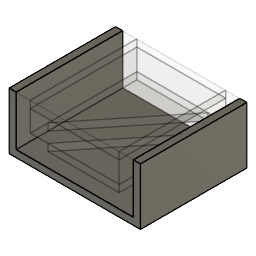
V4.3 (Autodesk Fusion 360 design; units mm, degrees)
part number: 2026-06-11-15-33-25-034
part number: 2026-06-11-15-44-55-864
part number: 2026-06-11-15-46-27-976
part number: 2026-06-11-15-51-44-010
part number: 2026-06-11-15-55-50-120
part number: 2026-06-18-15-30-37-176
part number: 2026-06-18-15-32-28-771
part number: 2026-06-18-15-36-27-577
part number: 2026-06-18-15-36-38-430
part number: 2026-06-18-15-43-19-432
part number: 2026-06-18-15-44-30-441
Autodesk Fusion 360 part; units mm, degrees
sketch "Esquisse5" plane through (0, 0, 0) normal (0, 0, 1) x (1, 0, 0)
  line L0 (0, 0) -> (37, 0)
  line L1 (37, 0) -> (37, 30)
  line L2 (37, 30) -> (0, 30)
  line L3 (0, 30) -> (0, 0)
  line L4 (0, 30) -> (2, 30)
  line L5 (2, 30) -> (2, 0)
  line L6 (2, 0) -> (0, 0)
  line L7 (0, 0) -> (0, 30)
  dimension "d48" = 37
  dimension "d49" = 30
  dimension "d50" = 2
  dimension "d51" = 30
  constraint horizontal L0
  constraint vertical L1
  constraint horizontal L2
  constraint vertical L3
  constraint coincident L0.start L3.end
  constraint horizontal L4
  constraint vertical L5
  constraint horizontal L6
  constraint vertical L7
  measures "d48" distance of L0.start L0.end
  measures "d49" distance of L0.start L2.end
  measures "d50" distance of L2.end L4.end
  measures "d51" distance of L2.end L0.start
extrude "Extrusion1" add sketch "Esquisse5" along normal blind 2 contours L0 L1 L2 L5 makes body 1 in component "Shield"
sketch "Esquisse1" plane through (0, 0, 0) normal (0, 0, 1) x (1, 0, 0) in component "Shield"
  line L0 (2, 30) -> (0, 30)
  line L1 (0, 30) -> (0, 0)
  line L2 (0, 0) -> (2, 0)
  line L3 (2, 0) -> (2, 30)
  line L4 (35, 30) -> (37, 30)
  line L5 (37, 30) -> (37, 0)
  line L6 (37, 0) -> (35, 0)
  line L7 (35, 0) -> (35, 30)
  point P0 (37, 0)
  dimension "d54" = 2
  dimension "d55" = 30
  dimension "d56" = 2
  dimension "d57" = 30
  constraint horizontal L0
  constraint vertical L1
  constraint horizontal L2
  constraint vertical L3
  constraint horizontal L4
  constraint vertical L5
  constraint horizontal L6
  constraint vertical L7
  constraint coincident L5 P0
  measures "d54" distance of L0.start L0.end
  measures "d55" distance of L0.start L2.end
  measures "d56" distance of L4.start L4.end
  measures "d57" distance of L4.start L6.end
extrude "Extrusion2" add sketch "Esquisse1" along normal blind 16 bodies 1 in component "Shield"
sketch "Esquisse2" plane through (0, 0, 2) normal (0, 0, 1) x (-1, 0, 0) in component "Shield"
  line L0 (-2, -30) -> (-2, 0)
  line L1 (-2, 0) -> (-35, 0)
  line L2 (-35, 0) -> (-35, -30)
  line L3 (-35, -30) -> (-2, -30)
sketch "Esquisse1 (2)" plane through (0, 0, 2) normal (0, 0, 1) x (-1, 0, 0) in component "Support"
  line L0 (-2, 0) -> (-6, 0)
  line L1 (-6, 0) -> (-6, -30)
  line L2 (-6, -30) -> (-2, -30)
  line L3 (-2, -30) -> (-2, 0)
  line L4 (-35, -30) -> (-31, -30)
  line L5 (-31, -30) -> (-31, 0)
  line L6 (-31, 0) -> (-35, 0)
  line L7 (-35, 0) -> (-35, -30)
  point P0 (-37, 0)
  dimension "d60" = 4
  dimension "d61" = 4
  dimension "d62" = 30
  dimension "d86" = 2
  dimension "d87" = 2
  constraint horizontal L0
  constraint vertical L1
  constraint horizontal L2
  constraint vertical L3
  constraint horizontal L4
  constraint vertical L5
  constraint horizontal L6
  constraint vertical L7
  measures "d60" distance of L0.start L0.end
  measures "d61" distance of L4.start L4.end
  measures "d62" distance of L4.start L6.end
  measures "d86" distance of origin L0.start
  measures "d87" distance of L6.end P0
extrude "Extrusion1'" add sketch "Esquisse1 (2)" along normal blind 14 separate body makes body 2 at (2, 20, 6.6667) makes body 3 at (35, 10, 6.6667) in component "Support"
extrude "Extrusion2'" add sketch "Esquisse2" along normal blind 4 bodies 2 3 in component "Support"
sketch "Esquisse2 (2)" plane through (0, 0, 6) normal (0, 0, 1) x (-1, 0, 0) in component "Support"
  line L0 (-6, -30) -> (-6, 0)
  line L1 (-6, 0) -> (-31, 0)
  line L2 (-31, 0) -> (-31, -30)
  line L3 (-31, -30) -> (-6, -30)
sketch "Esquisse1 (3)" plane through (0, 0, 6) normal (0, 0, 1) x (-1, 0, 0) in component "Capteur2"
  line L0 (-6, -5) -> (-26, -30)
  line L1 (-6, -30) -> (-6, 0)
  line L2 (-31, -30) -> (-6, -30)
  point P0 (-6, -30)
  point P1 (-6, 0)
  dimension "d67" = 20
  dimension "d69" = 5
  constraint coincident L0.start L1
  constraint coincident L0.end L2
  measures "d67" distance of L0.end P0
  measures "d69" distance of L0.start L1.end
extrude "Extrusion1''" add sketch "Esquisse1 (3)" along normal blind 2 separate body makes body 4 in component "Capteur2"
sketch "Esquisse2 (3)" plane through (0, 0, 6) normal (0, 0, 1) x (-1, 0, 0) in component "Capteur2"
  line L0 (-11, 0) -> (-31, -25)
  line L1 (-31, 0) -> (-31, -30)
  line L2 (-6, 0) -> (-31, 0)
  point P0 (-31, 0)
  point P1 (-31, -30)
  dimension "d72" = 20
  dimension "d73" = 5
  constraint coincident L0.end L1
  constraint coincident L0.start L2
  measures "d72" distance of L0.start P0
  measures "d73" vertical distance of L0.end P1
extrude "Extrusion1'''" add sketch "Esquisse2 (3)" along normal blind 2 separate body makes body 5 in component "Capteur1"
extrude "Extrusion3" add sketch "Esquisse2 (2)" along normal blind 2 bodies 2 in component "Support"
copy_body "CopierCollerCorps1" bodies 5 4 makes body 6 makes body 7 in component "Support"
combine "Combiner1" operation cut target body 2 tool bodies 6 7 in component "Support"
extrude "Extrusion1''''" add 1 faces at (21, 20, 8) along direction (0, 0, 1) blind 6 separate body on bodies 2 makes body 8 in component "Mousse (1)"
extrude "Extrusion2''" add 1 faces at (24.3333, 8.3333, 8) along direction (0, 0, 1) blind 6 on bodies 5 bodies 8 in component "Mousse (1)"
extrude "Extrusion3'" add 1 faces at (12.6667, 21.6667, 8) along direction (0, 0, 1) blind 6 on bodies 4 bodies 8 in component "Mousse (1)"
extrude "Extrusion1'''''" add 1 faces at (22.6667, 10, 14) along direction (0, 0, 1) blind 2 separate body on bodies 8 makes body 9 in component "plateau (1)"
sketch "Esquisse1 (4)" plane through (0, 0, 6) normal (0, 0, 1) x (-1, 0, 0) in component "trianglee_1"
  line L0 (-16, 0) -> (-16, -30)
  line L1 (-16, -30) -> (-6, -30)
  line L2 (-6, -30) -> (-6, 0)
  line L3 (-6, 0) -> (-16, 0)
  spline S0 degree 5 poles (-6, 0) (-6.4, -1) (-7.2, -3) (-8.4, -6) (-10, -10) (-12, -15) (-13.6, -19) (-14.8, -22) (-15.6, -24) (-16, -25) knots 0 0 0 0 0 0 0.2 0.4 0.6 0.8 1 1 1 1 1 1
  dimension "d33" = 5
  dimension "d47" = 20
  constraint coincident L3 L2.end
  constraint coincident L0 S0.end
  measures "d33" distance of L0.end S0.end
extrude "Extrusion1''''''" [rolled back] along distance 2 taper angle 0 in component "trianglee_1"
sketch "Esquisse1 (5)" plane through (0, 0, 6) normal (0, 0, 1) x (-1, 0, 0) in component "triangle_2"
  line L0 (-16, 0) -> (-16, -30)
  line L1 (-16, -30) -> (-6, -30)
  line L2 (-6, -30) -> (-6, 0)
  line L3 (-6, 0) -> (-16, 0)
  spline S0 degree 5 poles (-6, -5) (-6.4, -6) (-7.2, -8) (-8.4, -11) (-10, -15) (-12, -20) (-13.6, -24) (-14.8, -27) (-15.6, -29) (-16, -30) knots 0 0 0 0 0 0 0.2 0.4 0.6 0.8 1 1 1 1 1 1
  dimension "d37" = 5
  dimension "d46" = 20
  constraint coincident L2 S0.start
  constraint coincident L1 L0.end
  measures "d37" distance of L2.end S0.start
extrude "Extrusion1'''''''" [rolled back] along distance 2 taper angle 0 in component "triangle_2"
sketch "Esquisse1 (6)" plane through (0, 0, 8) normal (0, 0, 1) x (-1, 0, 0) in component "Mousse"
  line L0 (-16, -30) -> (-6, -5)
  line L1 (-6, -5) -> (-6, 0)
  line L2 (-6, 0) -> (-16, -25)
  line L3 (-16, -25) -> (-16, -30)
  line L4 (-6, -30) -> (-16, -30)
  line L5 (-16, -30) -> (-16, 0)
  line L6 (-16, 0) -> (-6, 0)
  line L7 (-6, 0) -> (-6, -30)
  constraint horizontal L4
  constraint vertical L5
  constraint horizontal L6
  constraint vertical L7
extrude "Extrusion1''''''''" [rolled back] taper angle 0 in component "Mousse"
extrude "Extrusion1'''''''''" [rolled back] along distance 2 taper angle 0 in component "plateau"
component "Shield" placed x (1, 0, 0) y (0, 1, 0) z (0, 0, 1) at (0, 0, 0)
component "Support" placed x (1, 0, 0) y (0, 1, 0) z (0, 0, 1) at (0, 0, 0)
component "Capteur1" placed x (1, 0, 0) y (0, 1, 0) z (0, 0, 1) at (0, 0, 0)
component "Capteur2" placed x (1, 0, 0) y (0, 1, 0) z (0, 0, 1) at (0, 0, 0)
component "Mousse (1)" placed x (1, 0, 0) y (0, 1, 0) z (0, 0, 1) at (0, 0, 0)
component "plateau (1)" placed x (1, 0, 0) y (0, 1, 0) z (0, 0, 1) at (0, 0, 0)
equation "épaisseur_mousse = 6 mm"
equation "distance_bord = 4 mm"
equation "epaisseur = 2 mm"
equation "distance_plaques = 5 mm"
equation "Longueur = 30 mm"
equation "hauteur = distance_bord + 3 * epaisseur + épaisseur_mousse"
equation "largeur_base_triangle = 20 mm"
equation "largeur = 2 * distance_bord + 2 * epaisseur + distance_plaques + largeur_base_triangle"
equation "d33 = distance_plaques"
equation "d34 = epaisseur"
equation "d37 = distance_plaques"
equation "d38 = epaisseur"
equation "d42 = épaisseur_mousse"
equation "d44 = epaisseur"
equation "d46 = largeur_base_triangle"
equation "d47 = largeur_base_triangle"
equation "d48 = largeur"
equation "d49 = Longueur"
equation "d50 = epaisseur"
equation "d51 = Longueur"
equation "d52 = epaisseur"
equation "d54 = epaisseur"
equation "d55 = Longueur"
equation "d56 = epaisseur"
equation "d57 = Longueur"
equation "d58 = hauteur"
equation "d60 = distance_bord"
equation "d61 = distance_bord"
equation "d62 = Longueur"
equation "d63 = hauteur - epaisseur"
equation "d65 = distance_bord"
equation "d67 = largeur_base_triangle"
equation "d69 = distance_plaques"
equation "d70 = epaisseur"
equation "d72 = largeur_base_triangle"
equation "d73 = distance_plaques"
equation "d74 = epaisseur"
equation "d76 = epaisseur"
equation "d78 = épaisseur_mousse"
equation "d80 = épaisseur_mousse"
equation "d82 = épaisseur_mousse"
equation "d84 = epaisseur"
equation "d86 = epaisseur"
equation "d87 = epaisseur"
